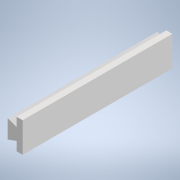
# Autodesk Inventor part: prismatic link outer
Saved by Autodesk Inventor 2021 (Build 250183000, 183)
## iProperties
Created: 2022-03-22
Part Number: prismatic link outer
Material: Generic
Document SubType Name: Modeling
Designer: techv
Density: 1 g/cm^3
Appearance: Default
Author: techv
Autodesk Inventor part; units mm, degrees
ref_plane "YZ Plane" through (0, 0, 0) normal (1, 0, 0) x (0, 1, 0)
ref_plane "XZ Plane" through (0, 0, 0) normal (0, 1, 0) x (-1, 0, 0)
sketch "Sketch1" plane through (0, 0, 0) normal (0, 0, 1) x (1, 0, 0)
  line L0 (-5, 10) -> (-5, -10) projected
  line L1 (-5, -10) -> (5, -10) projected
  line L2 (5, -10) -> (5, -4) projected
  line L3 (5, -4) -> (-1, -6.1838) projected
  line L4 (-1, -6.1838) -> (-1, 6.1838) projected
  line L5 (-1, 6.1838) -> (5, 4) projected
  line L6 (5, 4) -> (5, 10) projected
  line L7 (5, 10) -> (-5, 10) projected
  line L8 (-1, -10) -> (9, -10)
  line L9 (9, -10) -> (9, 10)
  line L10 (9, 10) -> (-1, 10)
  line L11 (-1, 10) -> (-1, -10)
  point P0 (0, 0)
  dimension "d0" = 10
  constraints: 8 end point, 2 parallel, 2 point on line, 1 horizontal, 1 perpendicular
  measures "d0" distance of L10.end L9.end
ref_plane "Work Plane1" through (-5, -10, -100) normal (0, 0, -1) x (0, 1, 0)
extrude "Extrusion1" add sketch "Sketch1" against normal up to surface (100 mm away) contours L10 L9 L8 L2 L3 L4 L5 L6
sketch "Sketch2" plane through (0, 0, 0) normal (0, 0, 1) x (1, 0, 0)
  line L0 (9, 10) -> (5, 10) projected
  line L1 (5, 10) -> (5, 4) projected
  line L2 (5, 4) -> (-1, 6.1838) projected
  line L3 (-1, 6.1838) -> (-1, -6.1838) projected
  line L4 (-1, -6.1838) -> (5, -4) projected
  line L5 (5, -4) -> (5, -10) projected
  line L6 (5, -10) -> (9, -10) projected
  line L7 (9, -10) -> (9, 10) projected
  line L8 (5, -10) -> (9, -10) projected
  line L9 (9, -10) -> (-5, -10)
  line L10 (-5, -10) -> (-5, 10)
  line L11 (-5, 10) -> (9, 10)
  line L12 (9, 10) -> (9, -10)
  point P0 (0, 0)
  dimension "d3" = 14
  dimension "d4" = 20
  constraints: 8 end point, 2 parallel, 1 horizontal, 1 perpendicular
  measures "d3" distance of L10.end L11.end
  measures "d4" distance of L9.end L10.end
extrude "Extrusion2" add sketch "Sketch2" along normal blind 3
sketch "Sketch3" plane through (9, -10, -100) normal (1, 0, 0) x (0, 0, -1)
  line L0 (-100, 16.1838) -> (-100, 3.8162) projected
  circle A0 centre (-94, 10) radius 1.5
  line L1 (0, 0) -> (-103, 0) projected
  circle A1 centre (-86, 10) radius 1.5
  circle A2 centre (-78, 10) radius 1.5
  circle A3 centre (-70, 10) radius 1.5
  circle A4 centre (-62, 10) radius 1.5
  circle A5 centre (-54, 10) radius 1.5
  circle A6 centre (-46, 10) radius 1.5
  circle A7 centre (-38, 10) radius 1.5
  circle A8 centre (-30, 10) radius 1.5
  circle A9 centre (-22, 10) radius 1.5
  circle A10 centre (-14, 10) radius 1.5
  circle A11 centre (-6, 10) radius 1.5
  point P0 (-100, 10)
  dimension "d7" = 3
  dimension "d8" = 6
  dimension "d11" = 8
  constraints: 12 centre point, 1 horizontal, 22 other
  measures "d7" diameter of A0
  measures "d8" distance from line of L0 A0.centre
  measures "d11" distance of A0.centre A1.centre
extrude "Extrusion3" cut sketch "Sketch3" against normal through all
sketch "Sketch4" plane through (0, 0, 3) normal (0, 0, 1) x (1, 0, 0)
  line L0 (-5, 10) -> (-5, -10) projected
  line L1 (-5, 10) -> (9, -10)
  line L2 (9, 10) -> (5, 10) projected
  line L3 (9, -10) -> (9, 10)
  line L4 (-5, -10) -> (5, -10) projected
  line L5 (9, 10) -> (-5, -10)
  line L6 (-0.75, -2.75) -> (4.75, -2.75)
  line L7 (4.75, -2.75) -> (4.75, 2.75)
  line L8 (4.75, 2.75) -> (-0.75, 2.75)
  line L9 (-0.75, 2.75) -> (-0.75, -2.75)
  line L10 (-0.75, -2.75) -> (4.75, 2.75) construction
  line L11 (4.75, -2.75) -> (-0.75, 2.75) construction
  point P0 (0, 0)
  point P1 (2, 0)
  dimension "d18" = 5.5
  dimension "d19" = 5.5
  constraints: 18 end point, 3 midpoint, 2 parallel, 2 perpendicular, 1 horizontal
  measures "d18" distance of L8.end L7.end
  measures "d19" distance of L7.end L6.end
extrude "Extrusion4" add sketch "Sketch4" along normal blind 7 contours L8 L5 L1 | L1 L5 L6 L9 L8 | L5 L1 L6 | L5 L8 L7 L6 L1
body "Solid1"
